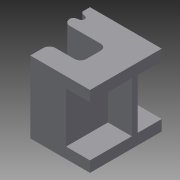
# Autodesk Inventor part: Hook2
Saved by Autodesk Inventor 2015 (Build 190159000, 159)
## iProperties
Created: 2015-01-19
Part Number: Hook2
Material: Generic
Document SubType Name: Modeling
Designer: nilesstanton
Density: 1 g/cm^3
Appearance: Default
Author: nilesstanton
Autodesk Inventor part; units mm, degrees
ref_plane "YZ Plane" through (0, 0, 0) normal (1, 0, 0) x (0, 1, 0)
ref_plane "XZ Plane" through (0, 0, 0) normal (0, 1, 0) x (-1, 0, 0)
ref_plane "XY Plane" through (0, 0, 0) normal (0, 0, 1) x (1, 0, 0)
sketch "Sketch1" plane through (0, 0, 0) normal (0, 1, 0) x (-1, 0, 0)
  line L0 (0, 0) -> (0, 76.2)
  line L1 (0, 0) -> (76.2, 0)
  line L2 (30.48, 27.94) -> (76.2, 27.94)
  line L3 (76.2, 27.94) -> (76.2, 18.415)
  line L4 (76.2, 0) -> (76.2, 9.525)
  line L5 (76.2, 18.415) -> (57.15, 13.97)
  line L6 (57.15, 13.97) -> (76.2, 9.525)
  line L7 (63.5, 76.2) -> (63.5, 55.88)
  line L8 (63.5, 55.88) -> (30.48, 55.88)
  line L9 (30.48, 55.88) -> (30.48, 27.94)
  line L10 (63.5, 76.2) -> (0, 76.2)
  dimension "d4" = 9.525
  dimension "d6" = 19.05
  dimension "d35" = 76.2
  dimension "d37" = 27.94
  dimension "d38" = 76.2
  dimension "d39" = 63.5
  dimension "d40" = 27.94
  dimension "d41" = 30.48
  constraints: 22 end point, 4 vertical, 2 equal length, 2 horizontal, 1 collinear, 1 parallel, 1 perpendicular
  measures "d4" distance of L1.end L4.end
  measures "d6" horizontal distance of L3.end L5.end
  measures "d35" distance of L0.start L0.end
  measures "d37" distance between parallel lines of L2 L8
  measures "d38" distance of L0.start L1.end
  measures "d39" distance of L7.start L0.end
  measures "d40" distance between parallel lines of L1 L2
  measures "d41" distance between parallel lines of L0 L9
extrude "Extrusion1" add sketch "Sketch1" along normal blind 76.2
fillet "Fillet1" radius 6.35 1 edges at (-76.2, 38.1, 27.94)
fillet "Fillet2" radius 3.175 1 edges at (-57.15, 38.1, 13.97)
fillet "Fillet3" radius 3.175 1 edges at (-76.2, 38.1, 18.415)
fillet "Fillet4" radius 3.175 1 edges at (-76.2, 38.1, 9.525)
fillet "Fillet5" radius 6.35 1 edges at (-63.5, 38.1, 55.88)
fillet "Fillet6" radius 6.35 1 edges at (-30.48, 38.1, 27.94)
fillet "Fillet7" radius 6.35 1 edges at (-30.48, 38.1, 55.88)
sketch "Sketch4" plane through (-63.5, 0, 76.2) normal (0, 0, 1) x (1, 0, 0)
  line L0 (63.5, 11.43) -> (38.1, 11.43)
  line L1 (38.1, 11.43) -> (38.1, 64.77)
  line L2 (38.1, 64.77) -> (63.5, 64.77)
  line L3 (63.5, 64.77) -> (63.5, 11.43)
  line L4 (63.5, 0) -> (0, 0) projected
  line L5 (63.5, 76.2) -> (0, 76.2) construction
  line L6 (63.5, 0) -> (63.5, 76.2) projected
  dimension "d42" = 53.34
  dimension "d43" = 25.4
  dimension "d44" = 11.43
  dimension "d45" = 0
  constraints: 10 end point, 2 horizontal, 2 parallel, 1 perpendicular
  measures "d42" distance of L0.end L1.end
  measures "d43" distance of L0.start L0.end
  measures "d44" distance between parallel lines of L0 L4
  measures "d45" distance between parallel lines of L6 L3
extrude "Extrusion4" cut sketch "Sketch4" against normal blind 44.45
sketch "Sketch5" plane through (0, 0, 76.2) normal (1, 0, 0) x (0, 0, -1)
  line L0 (76.2, 11.43) -> (50.8, 11.43)
  line L1 (50.8, 11.43) -> (50.8, 64.77)
  line L2 (50.8, 64.77) -> (76.2, 64.77)
  line L3 (76.2, 64.77) -> (76.2, 11.43)
  line L4 (76.2, 0) -> (76.2, 76.2) projected
  line L5 (0, 76.2) -> (76.2, 76.2) projected
  dimension "d48" = 53.34
  dimension "d49" = 25.4
  dimension "d50" = 0
  dimension "d51" = 11.43
  constraints: 8 end point, 2 parallel, 1 horizontal, 1 perpendicular
  measures "d48" distance of L0.end L1.end
  measures "d49" distance of L0.start L0.end
  measures "d50" distance between parallel lines of L3 L4
  measures "d51" distance between parallel lines of L5 L2
extrude "Extrusion5" cut sketch "Sketch5" against normal blind 50.8
body "Solid1"
